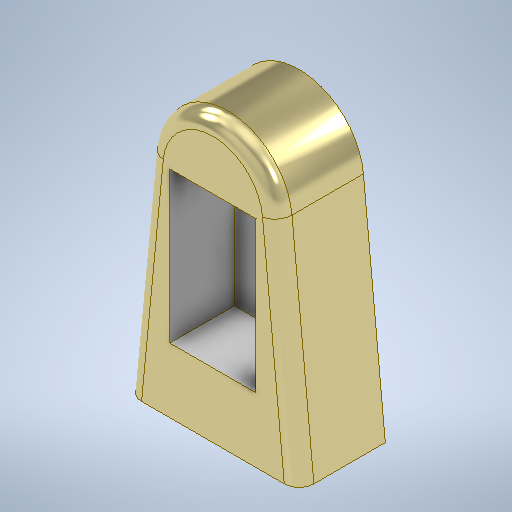
# Autodesk Inventor part: Robot_arm_3
Saved by Autodesk Inventor 2025 (Build 290162010, 162A)
## iProperties
Created: 2024-07-13
Part Number: Robot_arm_3
Material: Generic
Document SubType Name: Modeling
Designer: saees
Density: 1 g/cm^3
Appearance: Gold - Metal
Author: saees
Autodesk Inventor part; units mm, degrees
ref_plane "YZ Plane" through (0, 0, 0) normal (1, 0, 0) x (0, 1, 0)
ref_plane "XZ Plane" through (0, 0, 0) normal (0, 1, 0) x (-1, 0, 0)
ref_plane "XY Plane" through (0, 0, 0) normal (0, 0, 1) x (1, 0, 0)
sketch "Sketch1" plane through (0, 0, 0) normal (0, 0, 1) x (1, 0, 0)
  arc A0 (29.8554, 102.9422) -> (-29.8554, 102.9422) centre (0, 100) ccw
  line L0 (-29.8554, 102.9422) -> (-40, 0)
  line L1 (-40, 0) -> (40, 0)
  line L2 (40, 0) -> (29.8554, 102.9422)
  point P0 (0, 0)
  point P1 (0, 0)
  dimension "d0" = 80
  dimension "d1" = 60
  dimension "d2" = 100
  constraints: 6 end point, 2 point on circle, 2 tangent, 1 centre point, 1 coincident, 1 horizontal, 1 midpoint, 1 vertical alignment
  measures "d0" distance of L0.end L1.end
  measures "d1" diameter of A0
  measures "d2" distance of point (0, 0) A0.centre
extrude "Extrusion1" add sketch "Sketch1" along normal blind 40
sketch "Sketch2" plane through (0, 0, 40) normal (0, 0, 1) x (1, 0, 0)
  line L0 (-20, 100) -> (20, 100)
  line L1 (20, 100) -> (20, 30)
  line L2 (20, 30) -> (-20, 30)
  line L3 (-20, 30) -> (-20, 100)
  line L4 (-40, 0) -> (40, 0) projected
  arc A0 (29.8554, 102.9422) -> (-29.8554, 102.9422) centre (0, 100) ccw projected
  point P0 (0, 0)
  point P1 (0, 100)
  point P2 (0, 0)
  point P3 (0, 130)
  dimension "d5" = 70
  dimension "d6" = 40
  dimension "d7" = 30
  constraints: 8 end point, 2 midpoint, 2 parallel, 1 horizontal, 1 perpendicular, 1 point on circle, 1 vertical alignment
  measures "d5" distance of L2.end L0.start
  measures "d6" distance of L0.start L0.end
  measures "d7" distance of point (0, 130) point (0, 100)
extrude "Extrusion2" cut sketch "Sketch2" against normal blind 30
fillet "Fillet1" radius 6.858 3 edges at (0, 130, 40) (-34.9277, 51.4711, 40) (34.9277, 51.4711, 40)
sketch "Sketch3" plane through (-40, 0, 0) normal (0, -1, 0) x (1, 0, 0)
  line L0 (0, 0) -> (80, 0) projected
  line L1 (80, 0) -> (80, 33.142) projected
  line L2 (6.8912, 40) -> (73.1088, 40) projected
  circle A0 centre (40, 16.571) radius 2.5
  point P0 (40, 0)
  point P1 (40, 40)
  point P2 (80, 16.571)
  dimension "d11" = 5
  constraints: 2 midpoint, 1 centre point, 1 horizontal alignment, 1 vertical alignment
  measures "d11" diameter of A0
extrude "Extrusion3" cut sketch "Sketch3" against normal blind 30
sketch "Sketch4" plane through (0, 0, 10) normal (0, 0, 1) x (1, 0, 0)
  circle A0 centre (0, 80) radius 2.5
  line L0 (20, 30) -> (-20, 30) projected
  line L1 (20, 100) -> (20, 30) projected
  line L2 (-20, 100) -> (20, 100) projected
  line L3 (-20, 30) -> (-20, 100) projected
  point P0 (0, 0)
  dimension "d14" = 20
  dimension "d15" = 5
  dimension "d16" = 20
  constraints: 1 centre point
  measures "d14" distance from line of L2 A0.centre
  measures "d15" diameter of A0
  measures "d16" horizontal distance of L2.start A0.centre
extrude "Extrusion4" cut sketch "Sketch4" against normal blind 30 contours A0
body "Solid1"
